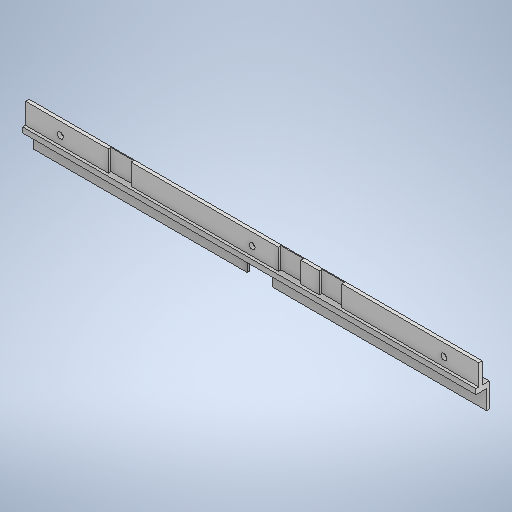
# Autodesk Inventor part: Lower mount
Saved by Autodesk Inventor 2025 (Build 290162000, 162)
## iProperties
Created: 2024-07-17
Part Number: Lower mount
Material: Generic
Document SubType Name: Modeling
Designer: adam
Density: 1 g/cm^3
Appearance: Default
Author: adam
Autodesk Inventor part; units mm, degrees
ref_plane "YZ Plane" through (0, 0, 0) normal (1, 0, 0) x (0, 1, 0)
ref_plane "XZ Plane" through (0, 0, 0) normal (0, 1, 0) x (-1, 0, 0)
ref_plane "XY Plane" through (0, 0, 0) normal (0, 0, 1) x (1, 0, 0)
sketch "Sketch1" plane through (0, 0, 0) normal (0, 0, 1) x (1, 0, 0)
  circle A0 centre (0, 0) radius 1.75
  circle A1 centre (110, 0) radius 1.75
  circle A2 centre (-110, 0) radius 1.75
  line L0 (-130, 7) -> (130, 7)
  line L1 (130, 7) -> (130, -5)
  line L2 (130, -5) -> (-130, -5)
  line L3 (-130, -5) -> (-130, 7)
  dimension "d0" = 3.5
  dimension "d1" = 110
  dimension "d2" = 110
  dimension "d3" = 130
  dimension "d4" = 130
  dimension "d5" = 7
  dimension "d6" = 5
  constraints: 8 end point, 3 centre point, 2 equal radius, 2 horizontal alignment, 2 parallel, 1 coincident, 1 horizontal, 1 perpendicular
  measures "d0" diameter of A0
  measures "d1" distance of point (0, 0) A2.centre
  measures "d2" distance of A1.centre point (0, 0)
  measures "d3" distance from line of L3 point (0, 0)
  measures "d4" distance from line of point (0, 0) L1
  measures "d5" distance from line of L0 point (0, 0)
  measures "d6" distance from line of L2 point (0, 0)
extrude "Extrusion1" add sketch "Sketch1" along normal blind 2
sketch "Sketch2" plane through (-130, -5, 0) normal (0, -1, 0) x (1, 0, 0)
  line L0 (0, 0) -> (260, 0) projected
  line L1 (0, 0) -> (260, 0)
  line L2 (260, 0) -> (260, 3.6)
  line L3 (260, 3.6) -> (0, 3.6)
  line L4 (0, 3.6) -> (0, 0)
  line L5 (260, 0) -> (260, 2) projected
  line L6 (0, 2) -> (260, 2) projected
  point P0 (130, 0)
  dimension "d9" = 1.6
  constraints: 8 end point, 2 parallel, 1 collinear, 1 horizontal, 1 perpendicular
  measures "d9" distance between parallel lines of L3 L6
extrude "Extrusion2" add sketch "Sketch2" along normal blind 3
sketch "Sketch3" plane through (0, 0, 0) normal (0, 0, -1) x (-1, 0, 0)
  line L0 (130, -5) -> (-130, -5) projected
  line L1 (130, -5) -> (130, -8) projected
  line L2 (130, -5) -> (130, -8)
  line L3 (130, -8) -> (-130, -8)
  line L4 (-130, -8) -> (-130, -5)
  point P0 (0, 0)
  constraints: 6 end point, 2 perpendicular, 1 collinear
extrude "Extrusion3" add sketch "Sketch3" along normal blind 4
sketch "Sketch4" plane through (-130, -8, 0) normal (0, -1, 0) x (1, 0, 0)
  line L0 (260, -4) -> (0, -4) projected
  line L1 (0, 0) -> (0, -4) projected
  line L2 (0, -4) -> (0, -2.5)
  line L3 (0, -2.5) -> (260, -2.5)
  line L4 (260, 0) -> (260, -4) projected
  line L5 (260, -2.5) -> (260, -4)
  point P0 (130, 0)
  dimension "d14" = 1.5
  constraints: 6 end point, 2 point on line, 1 collinear, 1 horizontal
  measures "d14" distance between parallel lines of L0 L3
extrude "Extrusion4" add sketch "Sketch4" along normal blind 11
sketch "Sketch5" plane through (0, 0, 2) normal (0, 0, 1) x (1, 0, 0)
  line L0 (130, 7) -> (-130, 7) projected
  line L1 (-82.5, 7) -> (-69.5, 7)
  line L2 (-69.5, 7) -> (-69.5, -5)
  line L3 (-69.5, -5) -> (-82.5, -5)
  line L4 (-82.5, -5) -> (-82.5, 7)
  line L5 (15, 7) -> (28, 7)
  line L6 (28, 7) -> (28, -5)
  line L7 (28, -5) -> (15, -5)
  line L8 (15, -5) -> (15, 7)
  line L9 (38.5, 7) -> (51.5, 7)
  line L10 (51.5, 7) -> (51.5, -5)
  line L11 (51.5, -5) -> (38.5, -5)
  line L12 (38.5, -5) -> (38.5, 7)
  line L13 (-130, -5) -> (130, -5) projected
  point P0 (0, 0)
  point P1 (-76, -5)
  point P2 (21.5, -5)
  point P3 (45, -5)
  dimension "d17" = 13
  dimension "d19" = 76
  dimension "d20" = 21.5
  dimension "d21" = 45
  constraints: 24 end point, 6 parallel, 4 equal length, 3 horizontal, 3 midpoint, 3 perpendicular, 3 point on line, 1 collinear
  measures "d17" distance of L2.end L3.end
  measures "d19" horizontal distance of point (0, 0) point (-76, -5)
  measures "d20" horizontal distance of point (21.5, -5) point (0, 0)
  measures "d21" horizontal distance of point (0, 0) point (45, -5)
extrude "Extrusion5" cut sketch "Sketch5" against normal blind 1.5 contours L10 L11 L12 L0 | L6 L7 L8 L0 | L2 L3 L4 L0
sketch "Sketch6" plane through (-130, -8, -2.5) normal (0, 0, 1) x (1, 0, 0)
  circle A0 centre (130, 8) radius 1.75 construction
  line L0 (130, 8) -> (130, -11) construction
  line L1 (1, -11) -> (259, -11) construction
  line L2 (122.75, -11) -> (137.25, -11)
  line L3 (137.25, -11) -> (137.25, -3)
  line L4 (137.25, -3) -> (122.75, -3)
  line L5 (122.75, -3) -> (122.75, -11)
  point P0 (130, -3)
  dimension "d25" = 14.5
  dimension "d26" = 8
  constraints: 10 end point, 2 midpoint, 2 parallel, 2 point on line, 1 horizontal, 1 perpendicular
  measures "d25" distance of L3.end L4.end
  measures "d26" distance of L2.end L3.end
extrude "Extrusion6" cut sketch "Sketch6" against normal up to surface (1.5 mm away)
equation "\"d2\" = d1"
equation "\"d4\" = d3"
body "Solid1"
